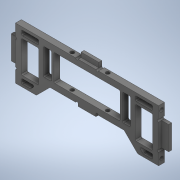
# Autodesk Inventor part: Trunk_chest_frame
Saved by Autodesk Inventor 2020.4 (Build 244396000, 396)
## iProperties
Created: 2022-01-02
Part Number: Trunk_chest_frame
Material: アセタール樹脂、黒
Document SubType Name: Modeling
Designer: Masato Kubotera
Density: 1.425 g/cm^3
Appearance: 滑らか - 黒
Mass: 13.4757 g
Surface Area: 93.011 cm^2
Volume: 9.45666 cm^3
Author: Masato Kubotera
Autodesk Inventor part; units mm, degrees
ref_plane "YZ Plane" through (0, 0, 0) normal (1, 0, 0) x (0, 1, 0)
ref_plane "XZ Plane" through (0, 0, 0) normal (0, 1, 0) x (-1, 0, 0)
ref_plane "XY Plane" through (0, 0, 0) normal (0, 0, 1) x (1, 0, 0)
sketch "スケッチ1" plane through (0, 0, 0) normal (0, 0, 1) x (1, 0, 0)
  line L0 (-60.5, 22) -> (60.5, 22) construction
  line L1 (60.5, 22) -> (60.5, -22) construction
  line L2 (60.5, -22) -> (-60.5, -22) construction
  line L3 (-60.5, -22) -> (-60.5, 22) construction
  line L4 (-60.5, 22) -> (60.5, -22) construction
  line L5 (60.5, 22) -> (-60.5, -22) construction
  line L6 (-60.5, 0) -> (60.5, 0) construction
  line L7 (-60.5, 5.75) -> (60.5, 5.75) construction
  line L8 (0, 22) -> (0, -22) construction
  line L9 (-60.5, 0) -> (60.5, 0) construction
  line L10 (7.5, 26) -> (-7.5, 26)
  line L11 (-7.5, 26) -> (-7.5, 22)
  arc A0 (-9.6, 22) -> (-7.5, 22) centre (-8.55, 22) ccw
  line L12 (-16, 22) -> (-16, -10.5) construction
  line L13 (-60.5, -10.5) -> (60.5, -10.5) construction
  line L14 (7.5, 26) -> (7.5, 22)
  arc A1 (7.5, 22) -> (9.6, 22) centre (8.55, 22) ccw
  line L15 (16, 22) -> (16, -10.5) construction
  line L16 (-60.5, 16) -> (60.5, 16) construction
  line L17 (-30, 16) -> (-30, -16) construction
  line L18 (-41.8, 16) -> (-41.8, -16) construction
  line L19 (-60.5, -16) -> (60.5, -16) construction
  line L20 (-54.5, 13.5) -> (-41.8, 13.5)
  line L21 (-40.8, 12.5) -> (-40.8, -12.5)
  line L22 (-41.8, -13.5) -> (-54.5, -13.5)
  line L23 (-55.5, -12.5) -> (-55.5, 12.5)
  line L24 (-55.5, 13.5) -> (-40.8, -13.5) construction
  line L25 (-40.8, 13.5) -> (-55.5, -13.5) construction
  arc A2 (-54.5, 13.5) -> (-55.5, 12.5) centre (-54.5, 12.5) ccw
  arc A3 (-55.5, -12.5) -> (-54.5, -13.5) centre (-54.5, -12.5) ccw
  arc A4 (-41.8, -13.5) -> (-40.8, -12.5) centre (-41.8, -12.5) ccw
  arc A5 (-40.8, 12.5) -> (-41.8, 13.5) centre (-41.8, 12.5) ccw
  arc A6 (-7.5, -10.5) -> (-9.6, -10.5) centre (-8.55, -10.5) ccw
  arc A7 (9.6, -10.5) -> (7.5, -10.5) centre (8.55, -10.5) ccw
  line L26 (-9.6, -10.5) -> (-31.3147, -10.5)
  line L27 (-60.5, -22) -> (-42.8147, -22)
  line L28 (-60.5, 22) -> (-9.6, 22)
  line L29 (-54.5, 19.75) -> (-41.8, 19.75)
  line L30 (-40.8, 18.75) -> (-40.8, 16.75)
  line L31 (-41.8, 15.75) -> (-54.5, 15.75)
  line L32 (-55.5, 16.75) -> (-55.5, 18.75)
  line L33 (-55.5, 19.75) -> (-40.8, 15.75) construction
  line L34 (-40.8, 19.75) -> (-55.5, 15.75) construction
  line L35 (-30, 22) -> (-30, 26) construction
  line L36 (-30, 26) -> (30, 26) construction
  line L37 (30, 26) -> (30, 22) construction
  line L38 (30, 22) -> (-30, 26) construction
  line L39 (-30, 22) -> (30, 26) construction
  line L40 (-28, 26) -> (-28, -16) construction
  line L41 (-7.5, -10.5) -> (-7.5, -12.5)
  line L42 (-7.5, -12.5) -> (7.5, -12.5)
  line L43 (7.5, -10.5) -> (7.5, -12.5)
  line L44 (-7.5, -12.5) -> (-28, -12.5) construction
  line L45 (-60.5, 10) -> (-66.5, 10)
  line L46 (-66.5, 10) -> (-66.5, -10)
  line L47 (-60.5, -10) -> (-66.5, -10)
  arc A8 (-60.5, 10) -> (-60.5, 12.1) centre (-60.5, 11.05) ccw
  arc A9 (-60.5, -12.1) -> (-60.5, -10) centre (-60.5, -11.05) ccw
  line L48 (-60.5, 22) -> (-60.5, 12.1)
  line L49 (-60.5, -12.1) -> (-60.5, -22)
  arc A10 (-54.5, 19.75) -> (-55.5, 18.75) centre (-54.5, 18.75) ccw
  arc A11 (-55.5, 16.75) -> (-54.5, 15.75) centre (-54.5, 16.75) ccw
  arc A12 (-40.8, 18.75) -> (-41.8, 19.75) centre (-41.8, 18.75) ccw
  arc A13 (-41.8, 15.75) -> (-40.8, 16.75) centre (-41.8, 16.75) ccw
  line L50 (-55.5, 17.75) -> (-60.5, 17.75) construction
  line L51 (-60.5, 15.75) -> (-56.5, 15.75) construction
  line L52 (-60.5, 19.75) -> (-56.5, 19.75) construction
  line L53 (-54.5, -19.75) -> (-48.05, -19.75)
  arc A14 (-55.5, -18.75) -> (-54.5, -19.75) centre (-54.5, -18.75) ccw
  arc A15 (-54.5, -15.75) -> (-55.5, -16.75) centre (-54.5, -16.75) ccw
  line L54 (-55.5, -17.75) -> (-60.5, -17.75) construction
  line L55 (-60.5, -15.75) -> (-56.5, -15.75) construction
  line L56 (-60.5, -19.75) -> (-56.5, -19.75) construction
  line L57 (-55.5, -16.75) -> (-55.5, -18.75)
  line L58 (0, 26) -> (0, -12.5)
  line L59 (-60.5, 10) -> (-60.5, -10)
  line L60 (-7.5, 22) -> (7.5, 22)
  line L61 (-35.8, 17) -> (-31, 17)
  line L62 (-30, 16) -> (-30, -4.5)
  line L63 (-31, -5.5) -> (-35.8, -5.5)
  line L64 (-36.8, 17) -> (-30, -5.5) construction
  line L65 (-30, 17) -> (-36.8, -5.5) construction
  arc A16 (-35.8, 17) -> (-36.8, 16) centre (-35.8, 16) ccw
  arc A17 (-30, 16) -> (-31, 17) centre (-31, 16) ccw
  arc A18 (-31, -5.5) -> (-30, -4.5) centre (-31, -4.5) ccw
  arc A19 (-36.8, -4.5) -> (-35.8, -5.5) centre (-35.8, -4.5) ccw
  line L66 (27, 17) -> (-27, 17)
  line L67 (-28, 16) -> (-28, -4.5)
  line L68 (-27, -5.5) -> (27, -5.5)
  line L69 (28, -4.5) -> (28, 16)
  line L70 (28, 17) -> (-28, -5.5) construction
  line L71 (-28, 17) -> (28, -5.5) construction
  arc A20 (-27, 17) -> (-28, 16) centre (-27, 16) ccw
  arc A21 (-28, -4.5) -> (-27, -5.5) centre (-27, -4.5) ccw
  arc A22 (27, -5.5) -> (28, -4.5) centre (27, -4.5) ccw
  arc A23 (28, 16) -> (27, 17) centre (27, 16) ccw
  line L72 (-36.8, 16) -> (-36.8, -4.5)
  line L73 (-42.8147, -22) -> (-31.3147, -10.5)
  line L74 (-45.3429, -17.4571) -> (-47.3429, -19.4571)
  line L75 (-46.05, -15.75) -> (-54.5, -15.75)
  arc A24 (-45.3429, -17.4571) -> (-46.05, -15.75) centre (-46.05, -16.75) ccw
  arc A25 (-48.05, -19.75) -> (-47.3429, -19.4571) centre (-48.05, -18.75) ccw
  point P0 (0, 0)
  point P1 (-48.15, 0)
  point P2 (-48.15, 17.75)
  point P3 (0, 24)
  point P4 (0, 24)
  point P5 (0, 22)
  point P6 (-33.4, 5.75)
  point P7 (0, 5.75)
  point P8 (0, -5.5)
  point P9 (0, 17)
  dimension "d0" = 121
  dimension "d3" = 16.25
  dimension "d4" = 1.05
  dimension "d5" = 32.5
  dimension "d6" = 32
  dimension "d7" = 15
  dimension "d8" = 4
  dimension "d11" = 30.5
  dimension "d12" = 11.8
  dimension "d13" = 32
  dimension "d14" = 16
  dimension "d15" = 6
  dimension "d16" = 1
  dimension "d18" = 1
  dimension "d19" = 5
  dimension "d20" = 5.5
  dimension "d21" = 6
  dimension "d26" = 27
  dimension "d29" = 4
  dimension "d30" = 2
  dimension "d31" = 2
  dimension "d32" = 1.05
  dimension "d33" = 6
  dimension "d34" = 20
  dimension "d35" = 8.5
  dimension "d36" = 4.25
  dimension "d37" = 1
  dimension "d38" = 4
  dimension "d39" = 35.5
  dimension "d67" = 44
  dimension "d81" = 1
  dimension "d87" = 1
  dimension "d88" = 5
  dimension "d90" = 4
  dimension "d91" = 2
  dimension "d98" = 2
  dimension "d99" = 5.75
  dimension "d100" = 5
  dimension "d101" = 45
  dimension "d102" = 1
  constraints: 150 end point, 57 point on line, 52 point on circle, 37 tangent, 31 symmetric about line, 26 centre point, 21 midpoint, 16 perpendicular, 13 equal radius, 12 horizontal, 12 parallel, 8 collinear, 4 vertical, 18 other
  measures "d0" distance of L1.end L2.end
  measures "d3" distance of L7.start L0.start
  measures "d4" radius of A0
  measures "d5" distance of L13.start L0.start
  measures "d6" distance of L15.start L12.start
  measures "d7" distance of L10.start L10.end
  measures "d8" distance of L10.start L14.end
  measures "d11" distance of L16.start L17.start
  measures "d12" distance of L17.start L18.start
  measures "d13" distance of L16.start L19.start
  measures "d14" distance of L19.start L6.start
  measures "d15" distance of L2.end L19.start
  measures "d16" radius of A2
  measures "d18" distance between parallel lines of L21 L18
  measures "d19" distance from line of L0.start L23
  measures "d20" distance of L19.start L13.start
  measures "d21" distance of L16.start L0.start
  measures "d26" distance of L22.start L20.end
  measures "d29" distance of L34.start L33.end
  measures "d30" distance of L41.start L41.end
  measures "d31" distance of L35.end L40.start
  measures "d32" radius of A8
  measures "d33" distance of L45.end L45.start
  measures "d34" distance of L45.end L46.end
  measures "d35" vertical distance of L20.start L0.start
  measures "d36" vertical distance of L0.start point (-48.15, 17.75)
  measures "d37" radius of A10
  measures "d38" distance of L51.end L52.end
  measures "d39" distance of L54.end L50.end
  measures "d67" distance of L2.end L0.start
  measures "d81" radius of A16
  measures "d87" radius of A20
  measures "d88" distance between parallel lines of L66 L0
  measures "d90" distance between parallel lines of L21 L72
  measures "d91" distance between parallel lines of L67 L62
  measures "d98" horizontal distance of L35.start L67.start
  measures "d99" distance of L6.start L7.start
  measures "d100" distance between parallel lines of L74 L73
  measures "d101" angle of L73 L27
  measures "d102" radius of A24
extrude "押し出し1" add sketch "スケッチ1" along normal blind 5 contours L58 L66 A20 L67 A21 L68 L42 L41 A6 L26 L73 L27 L49 A9 L59 A8 L48 L28 A0 L60
extrude "押し出し2" add sketch "スケッチ1" along normal blind 2.5 contours L58 L60 L11 L10 | L59 L47 L46 L45
sketch "スケッチ2" plane through (-60.5, 12.1, 0) normal (-1, 0, 0) x (0, 0, 1)
  line L0 (2.5, 9.9) -> (2.5, -34.1)
  line L1 (0, -34.1) -> (5, -34.1) projected
  line L2 (0, -12.1) -> (5, -12.1)
  line L3 (0, 9.9) -> (5, 9.9) projected
  line L4 (5, -2.1) -> (5, -22.1) projected
  point P0 (2.5, 5.65)
  point P1 (2.5, -29.85)
  dimension "d42" = 35.5
  constraints: 4 end point, 3 midpoint, 2 point on line, 1 symmetric about line
  measures "d42" distance of point (2.5, -29.85) point (2.5, 5.65)
hole "穴1" at (-60.5, -17.75, 2.5) at (-60.5, 17.75, 2.5) direction (1, 0, 0) diameter 3.242 depth 5 tip angle 118 thread size "M4x0.7" class "6H" standard "ISO Metric profile"
sketch "スケッチ3" plane through (-60.5, 22, 0) normal (0, 1, 0) x (1, 0, 0)
  line L0 (0, 0) -> (0, -5) projected
  line L1 (0, -2.5) -> (60.5, -2.5)
  line L2 (0, 0) -> (0, -5) projected
  line L3 (60.5, 0) -> (60.5, -5) projected
  point P0 (45.5, -2.5)
  dimension "d94" = 15
  constraints: 2 end point, 2 midpoint, 1 horizontal, 1 point on line
  measures "d94" distance from line of L3 point (45.5, -2.5)
hole "穴2" at (-15, 22, 2.5) direction (0, -1, 0) diameter 3.242 depth 5 tip angle 118 thread size "M4x0.7" class "6H" standard "ISO Metric profile"
sketch "スケッチ4" plane through (-20, -10.5, 0) normal (0, -1, 0) x (1, 0, 0)
  circle A0 centre (5, 2.5) radius 1.621 projected
  point P0 (20, 0)
  point P1 (5, 2.5)
  constraints: 1 coincident
hole "穴3" at (-15, -10.5, 2.5) direction (0, 1, 0) diameter 3.242 depth 5 tip angle 118 thread size "M4x0.7" class "6H" standard "ISO Metric profile"
mirror "ミラー1" about plane through (0, -12.5, 0) normal (1, 0, 0)
fillet "フィレット2" radius 1 2 edges at (-42.8147, -22, 2.5) (-31.3147, -10.5, 2.5)
fillet "フィレット3" radius 2 1 edges at (42.8147, -22, 2.5)
equation "\"d3\" = 0.5 * d5"
equation "\"d14\" = 0.5 * d13"
equation "\"d18\" = d17"
equation "\"d32\" = d4"
equation "\"d17\" = 1"
